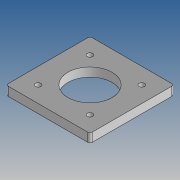
# Autodesk Inventor part: placa soporte motor
Saved by Autodesk Inventor 2017 (Build 210142000, 142)
## iProperties
Part Number: placa soporte motor
Material: Genérico
Document SubType Name: Modeling
Designer: Leo
Density: 1 g/cm^3
Appearance: Valor por defecto
Author: Leo
Autodesk Inventor part; units mm, degrees
ref_plane "YZ Plane" through (0, 0, 0) normal (1, 0, 0) x (0, 1, 0)
ref_plane "XZ Plane" through (0, 0, 0) normal (0, 1, 0) x (-1, 0, 0)
ref_plane "XY Plane" through (0, 0, 0) normal (0, 0, 1) x (1, 0, 0)
sketch "Boceto1" plane through (0, 0, 0) normal (0, 0, 1) x (1, 0, 0)
  line L0 (-36.2, 38.2) -> (36.2, 38.2)
  line L1 (38.2, 36.2) -> (38.2, -36.2)
  line L2 (36.2, -38.2) -> (-36.2, -38.2)
  line L3 (-38.2, -36.2) -> (-38.2, 36.2)
  arc A0 (-36.2, 38.2) -> (-38.2, 36.2) centre (-36.2, 36.2) ccw
  arc A1 (38.2, 36.2) -> (36.2, 38.2) centre (36.2, 36.2) ccw
  arc A2 (36.2, -38.2) -> (38.2, -36.2) centre (36.2, -36.2) ccw
  arc A3 (-38.2, -36.2) -> (-36.2, -38.2) centre (-36.2, -36.2) ccw
  line L4 (-36.2, 36.2) -> (36.2, -36.2) construction
  line L5 (-36.2, -36.2) -> (36.2, 36.2) construction
  circle A4 centre (23.55, 23.55) radius 2.5
  circle A5 centre (23.55, -23.55) radius 2.5
  circle A6 centre (-23.55, -23.55) radius 2.5
  circle A7 centre (-23.55, 23.55) radius 2.5
  circle A8 centre (0, 0) radius 20
  point P0 (-38.2, 38.2)
  point P1 (-38.2, -38.2)
  dimension "d0" = 76.4
  dimension "d1" = 2
  dimension "d2" = 5
  dimension "d3" = 61.6095
  dimension "d4" = 40
  dimension "d23" = 47.1
  constraints: 12 end point, 9 centre point, 8 point on circle, 8 point on line, 8 tangent, 6 equal radius, 2 coincident, 2 horizontal alignment, 2 parallel, 2 perpendicular, 2 vertical alignment, 1 horizontal, 1 midpoint
  measures "d0" distance of point (-38.2, -38.2) point (-38.2, 38.2)
  measures "d1" radius of A0
  measures "d2" diameter of A4
  measures "d4" diameter of A8
  measures "d23" distance of A6.centre A5.centre
extrude "Extrusión1" add sketch "Boceto1" against normal blind 8
